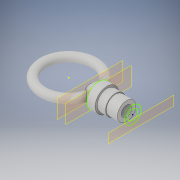
# Autodesk Inventor part: kims_perch2020
Saved by Autodesk Inventor 2018 (Build 220112000, 112)
## iProperties
Created: 2019-02-11
Part Number: kims_perch2020
Material: Generic
Document SubType Name: Modeling
Designer: Kim
Density: 1 g/cm^3
Appearance: Default
Author: Kim
Autodesk Inventor part; units mm, degrees
ref_plane "XZ Plane" through (0, 0, 0) normal (0, 1, 0) x (-1, 0, 0)
ref_plane "XY Plane" through (0, 0, 0) normal (0, 0, 1) x (1, 0, 0)
sketch "Sketch1" plane through (0, 0, 0) normal (0, 0, 1) x (1, 0, 0)
  circle A0 centre (-7.65, 0) radius 1.25
  line L0 (0, 4.1624) -> (0, -4.1624)
  point P0 (0, 0)
  dimension "d0" = 2.5
  constraints: 2 end point, 1 centre point, 1 vertical
  measures "d0" diameter of A0
revolve "Revolution1" add sketch "Sketch1" angle 360 about axis through (0, 4.1624, 0) along (0, -1, 0)
ref_plane "Work Plane1" through (21.6, 0, 0) normal (1, 0, 0) x (0, 1, 0)
sketch "Sketch2" plane through (21.6, 0, 0) normal (1, 0, 0) x (0, 1, 0)
  circle A0 centre (0, 0) radius 1.5
  circle A1 centre (0, 0) radius 2.5
  dimension "d3" = 3
  dimension "d4" = 5
  constraints: 2 centre point, 2 coincident
  measures "d3" diameter of A0
  measures "d4" diameter of A1
ref_plane "Work Plane2" through (8.9, 0, 0) normal (1, 0, 0) x (0, 1, 0)
sketch "Sketch3" plane through (8.9, 0, 0) normal (1, 0, 0) x (0, 1, 0)
  circle A0 centre (0, 0) radius 3.5297
  circle A1 centre (0, 0) radius 1.487
  constraints: 2 centre point, 2 coincident
extrude "Extrusion1" add sketch "Sketch3" along normal blind 2.54
extrude "Extrusion2" add sketch "Sketch2" against normal blind 2.54
sketch "Sketch5" plane through (11.44, 0, 0) normal (1, 0, 0) x (0, 0, -1)
  circle A0 centre (0, 0) radius 1.5
  circle A1 centre (0, 0) radius 2.9723
  constraints: 2 centre point, 2 coincident
sketch "Sketch6" plane through (19.06, 0, 0) normal (-1, 0, 0) x (0, 0, 1)
  circle A0 centre (0, 0) radius 2.5 projected
  circle A1 centre (0, 0) radius 1.5
  circle A2 centre (0, 0) radius 2.5
  constraints: 2 centre point, 2 coincident
sketch "Sketch7" plane through (0, 0, 0) normal (0, 1, 0) x (-1, 0, 0)
  point P0 (0, 0)
extrude "Extrusion3" add sketch "Sketch5" along normal blind 2.54
sketch "Sketch8" plane through (13.98, 0, 0) normal (1, 0, 0) x (0, 0, -1)
  circle A0 centre (0, 0) radius 1.487
  circle A1 centre (0, 0) radius 2.7524
  constraints: 2 centre point, 2 coincident
extrude "Extrusion4" add sketch "Sketch8" along normal blind 5.588
sketch "Sketch9" plane through (8.9, 0, 0) normal (1, 0, 0) x (0, 1, 0)
  circle A0 centre (0, 0) radius 3.5297
  constraints: 1 centre point, 1 coincident
ref_plane "Work Plane3" through (6.36, 0, 0) normal (1, 0, 0) x (0, 1, 0)
sketch "Sketch10" plane through (6.36, 0, 0) normal (1, 0, 0) x (0, 1, 0)
  circle A0 centre (0, 0) radius 1.578
  constraints: 1 centre point, 1 coincident
loft "Loft1" add profiles "Sketch10" section 2 edges at (8.9, -3.5297, 0)
sketch "Sketch11" plane through (21.6, 0, 0) normal (1, 0, 0) x (0, 1, 0)
  circle A0 centre (0, 0) radius 1.5635
  constraints: 1 centre point, 1 coincident
extrude "Extrusion5" cut sketch "Sketch11" against normal blind 12.7
sketch "Sketch12" plane through (21.6, 0, 0) normal (1, 0, 0) x (0, 1, 0)
  circle A0 centre (0, 0) radius 1.5635
  circle A1 centre (0, 0) radius 3.9487
  constraints: 2 centre point, 2 coincident
extrude "Extrusion6" cut sketch "Sketch12" against normal blind 4.318
body "Solid1"
